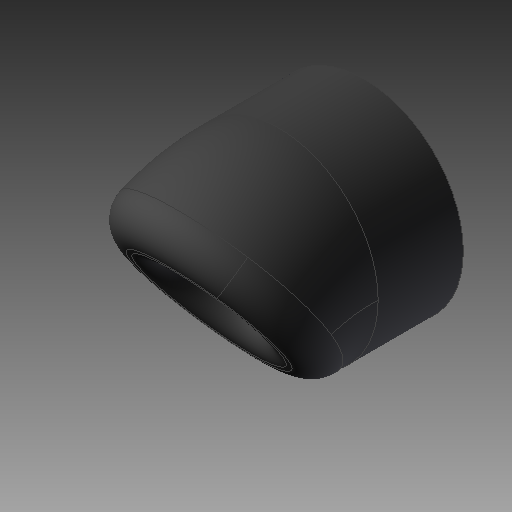
# Autodesk Inventor part: Eyes
Saved by Autodesk Inventor 2018 (Build 220112000, 112)
## iProperties
Created: 2018-03-03
Part Number: Eyes
Material: Generic
Document SubType Name: Modeling
Designer: reide
Density: 1 g/cm^3
Appearance: Default
Author: reide
Autodesk Inventor part; units mm, degrees
ref_plane "YZ Plane" through (0, 0, 0) normal (1, 0, 0) x (0, 1, 0)
ref_plane "XZ Plane" through (0, 0, 0) normal (0, 1, 0) x (-1, 0, 0)
ref_plane "XY Plane" through (0, 0, 0) normal (0, 0, 1) x (1, 0, 0)
sketch "Sketch1" plane through (0, 0, 0) normal (0, 0, 1) x (1, 0, 0)
  arc A0 (-4.9984, 0.1266) -> (-4.98, 0.4466) centre (0, 0) ccw projected
  circle A1 centre (0, 0) radius 7.5 projected
  circle A2 centre (0, 0) radius 7 projected
  circle A3 centre (0, 0) radius 7
  point P0 (0, 0)
  constraints: 1 centre point, 1 coincident, 1 concentric
extrude "Extrusion1" add sketch "Sketch1" along normal blind 6 contours A2
sketch "Sketch2" plane through (0, 0, 6) normal (0, 0, 1) x (1, 0, 0)
  line L0 (0, 0) -> (-2.839, 0)
  line L1 (-2.839, 0) -> (-2.839, 2.1073)
  line L2 (-2.839, 2.1073) -> (0, 2.1073)
  line L3 (0, 2.1073) -> (0, 0)
  constraints: 8 end point, 2 parallel, 1 horizontal, 1 perpendicular
extrude "Extrusion2" add sketch "Sketch2" along normal blind 1
sketch "Sketch3" plane through (0, 0, 6) normal (1, 0, 0) x (0, 0, -1)
  line L0 (0, 7) -> (0, -7) projected
  line L1 (0, 2.1073) -> (0, 0) projected
  line L2 (0, 0) -> (-1, 0) projected
  arc A0 (0, 0) -> (-5.1393, -1.322) centre (-0.5, -8.7067) ccw
  point P0 (6, 0)
  point P1 (-3.7243, -0.9054)
  point P2 (-4.3276, -1.2024)
  constraints: 3 point on circle, 1 centre point
sketch "Sketch4" plane through (0, 0, 6) normal (0, 0, 1) x (1, 0, 0)
  circle A0 centre (0, 0) radius 7
  circle A1 centre (0, 0) radius 2.65
  dimension "d20" = 5.3
  constraints: 2 centre point, 2 coincident
  measures "d20" diameter of A1
sketch "Sketch8" plane through (0, 0, 7) normal (0, 0, 1) x (1, 0, 0)
  circle A0 centre (0, 0) radius 2.65
  dimension "d17" = 5.3
  constraints: 1 centre point, 1 coincident
  measures "d17" diameter of A0
extrude "Extrusion3" cut sketch "Sketch8" against normal blind 100
sweep "Sweep6" add profiles "Sketch4" path "Sketch3" path curves A0
fillet "Fillet2" radius 2 2 edges at (-2.65, -1.322, 11.1393) (-7, -1.322, 11.1393)
body "Solid1"
